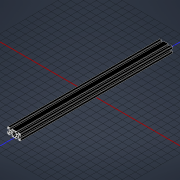
# Autodesk Inventor part: Extrusion_20x40x470
Saved by Autodesk Inventor 2022 (Build 260153000, 153)
## iProperties
Created: 2022-03-06
Part Number: Extrusion_20x40x470
Material: Aluminium 6061
Document SubType Name: Modeling
Designer: sleib
Density: 2.7 g/cm^3
Appearance: Eloxiert - Schwarz
Author: sleib
Autodesk Inventor part; units mm, degrees
ref_plane "YZ Plane" through (0, 0, 0) normal (1, 0, 0) x (0, 1, 0)
ref_plane "XZ Plane" through (0, 0, 0) normal (0, 1, 0) x (-1, 0, 0)
ref_plane "XY Plane" through (0, 0, 0) normal (0, 0, 1) x (1, 0, 0)
sketch "Skizze1" plane through (0, 0, 0) normal (0, 0, 1) x (1, 0, 0)
  circle A0 centre (10, 0) radius 2.56
  line L0 (10.5196, 4) -> (10, 3.7)
  line L1 (14, 0.5196) -> (14, 2.9393)
  line L2 (12.9393, 4) -> (10.5196, 4)
  line L3 (13.7, 0) -> (14, 0.5196)
  line L4 (14, 2.9393) -> (17.0607, 6)
  line L5 (17.0607, 6) -> (18, 6)
  line L6 (18, 6) -> (18, 3)
  line L7 (18, 3) -> (20, 3)
  line L8 (16, 7.0607) -> (12.9393, 4)
  line L9 (13, 8) -> (16, 8)
  line L10 (16, 8) -> (16, 7.0607)
  line L11 (20, 3) -> (20, 9)
  line L12 (19, 10) -> (13, 10)
  arc A1 (20, 9) -> (19, 10) centre (19, 9) ccw
  line L13 (13, 10) -> (13, 8)
  line L14 (10, 0) -> (19.7071, 9.7071) construction
  line L15 (-14.2899, 0) -> (14.2899, 0) construction
  line L16 (10, -14.2899) -> (10, 14.2899) construction
  line L17 (-28.2899, 0) -> (28.2899, 0) construction
  line L18 (0, -20.0059) -> (0, 20.0059) construction
  line L19 (14, -0.5196) -> (14, -2.9393)
  line L20 (13.7, 0) -> (14, -0.5196)
  circle A2 centre (10, 0) radius 2.56
  line L21 (10.5196, -4) -> (10, -3.7)
  line L22 (12.9393, -4) -> (10.5196, -4)
  line L23 (17.0607, -6) -> (18, -6)
  line L24 (14, -2.9393) -> (17.0607, -6)
  line L25 (16, -8) -> (16, -7.0607)
  line L26 (13, -8) -> (16, -8)
  line L27 (10, 0) -> (19.7071, -9.7071) construction
  line L28 (20, -3) -> (20, -9)
  line L29 (19, -10) -> (13, -10)
  arc A3 (19, -10) -> (20, -9) centre (19, -9) ccw
  line L30 (13, -10) -> (13, -8)
  line L31 (16, -7.0607) -> (12.9393, -4)
  line L32 (18, -3) -> (20, -3)
  line L33 (18, -6) -> (18, -3)
  line L34 (-14, 0.5196) -> (-14, 2.9393)
  line L35 (-13.7, 0) -> (-14, 0.5196)
  circle A4 centre (-10, 0) radius 2.56
  line L36 (-10.5196, 4) -> (-10, 3.7)
  line L37 (-12.9393, 4) -> (-10.5196, 4)
  line L38 (-17.0607, 6) -> (-18, 6)
  line L39 (-14, 2.9393) -> (-17.0607, 6)
  line L40 (-16, 8) -> (-16, 7.0607)
  line L41 (-13, 8) -> (-16, 8)
  line L42 (-10, 0) -> (-19.7071, 9.7071) construction
  line L43 (-10, -14.2899) -> (-10, 14.2899) construction
  line L44 (-20, 3) -> (-20, 9)
  line L45 (-19, 10) -> (-13, 10)
  arc A5 (-19, 10) -> (-20, 9) centre (-19, 9) ccw
  line L46 (-13, 10) -> (-13, 8)
  line L47 (-16, 7.0607) -> (-12.9393, 4)
  line L48 (-18, 3) -> (-20, 3)
  line L49 (-18, 6) -> (-18, 3)
  line L50 (-13.7, 0) -> (-14, -0.5196)
  line L51 (-14, -0.5196) -> (-14, -2.9393)
  line L52 (-10.5196, -4) -> (-10, -3.7)
  circle A6 centre (-10, 0) radius 2.56
  line L53 (-12.9393, -4) -> (-10.5196, -4)
  line L54 (-13, -10) -> (-13, -8)
  line L55 (-16, -7.0607) -> (-12.9393, -4)
  line L56 (-16, -8) -> (-16, -7.0607)
  line L57 (-13, -8) -> (-16, -8)
  line L58 (-14, -2.9393) -> (-17.0607, -6)
  line L59 (-10, 0) -> (-19.7071, -9.7071) construction
  line L60 (-19, -10) -> (-13, -10)
  line L61 (-17.0607, -6) -> (-18, -6)
  arc A7 (-20, -9) -> (-19, -10) centre (-19, -9) ccw
  line L62 (-20, -3) -> (-20, -9)
  line L63 (-18, -3) -> (-20, -3)
  line L64 (-18, -6) -> (-18, -3)
  line L65 (-9.4804, 4) -> (-10, 3.7)
  line L66 (-7.0607, -4) -> (-9.4804, -4)
  line L67 (-9.4804, -4) -> (-10, -3.7)
  line L68 (-7.0607, 4) -> (-9.4804, 4)
  line L69 (-4, 8) -> (-4, 7.0607)
  line L70 (-7, 8) -> (-4, 8)
  line L71 (-1, 10) -> (-7, 10)
  line L72 (-7, 10) -> (-7, 8)
  line L73 (-4, -7.0607) -> (-7.0607, -4)
  line L74 (-4, -8) -> (-4, -7.0607)
  line L75 (-1, -10) -> (-7, -10)
  line L76 (-7, -8) -> (-4, -8)
  line L77 (-7, -10) -> (-7, -8)
  line L78 (-4, 7.0607) -> (-7.0607, 4)
  line L79 (9.4804, 4) -> (10, 3.7)
  line L80 (7.0607, 4) -> (9.4804, 4)
  line L81 (4, 8) -> (4, 7.0607)
  line L82 (7, 8) -> (4, 8)
  line L83 (1, 10) -> (7, 10)
  line L84 (7, 10) -> (7, 8)
  line L85 (4, 7.0607) -> (7.0607, 4)
  line L86 (9.4804, -4) -> (10, -3.7)
  line L87 (7.0607, -4) -> (9.4804, -4)
  line L88 (7, -10) -> (7, -8)
  line L89 (4, -7.0607) -> (7.0607, -4)
  line L90 (4, -8) -> (4, -7.0607)
  line L91 (7, -8) -> (4, -8)
  line L92 (1, -10) -> (7, -10)
  line L93 (-1, 10) -> (1, 10)
  line L94 (-1, -10) -> (1, -10)
  line L95 (2.9393, 8) -> (-2.9393, 8)
  line L96 (2.9393, 8) -> (2.9393, 6)
  line L97 (6, 0.5196) -> (6, 2.9393)
  line L98 (6.3, 0) -> (6, 0.5196)
  line L99 (6, 2.9393) -> (2.9393, 6)
  line L100 (6.3, 0) -> (6, -0.5196)
  line L101 (6, -0.5196) -> (6, -2.9393)
  line L102 (6, -2.9393) -> (2.9393, -6)
  line L103 (-6.3, 0) -> (-6, -0.5196)
  line L104 (-6, 2.9393) -> (-2.9393, 6)
  line L105 (-6, 0.5196) -> (-6, 2.9393)
  line L106 (-6.3, 0) -> (-6, 0.5196)
  line L107 (-6, -0.5196) -> (-6, -2.9393)
  line L108 (-6, -2.9393) -> (-2.9393, -6)
  line L109 (-2.9393, 8) -> (-2.9393, 6)
  line L110 (2.9393, -6) -> (2.9393, -8)
  line L111 (2.9393, -8) -> (-2.9393, -8)
  line L112 (-2.9393, -8) -> (-2.9393, -6)
  point P0 (0, 0)
  point P1 (0, 8)
  dimension "d2" = 1.5
  dimension "d3" = 3
  dimension "d4" = 4
  dimension "d5" = 0.3
  dimension "d6" = 2
  dimension "d7" = 6
  dimension "d8" = 10
  dimension "d9" = 10
  dimension "d10" = 2
  dimension "d11" = 3
  dimension "d12" = 6
  dimension "d13" = 1
  dimension "d14" = 4
  dimension "d15" = 0.3
  dimension "d16" = 0.5196
  dimension "d17" = 0.5196
  dimension "d18" = 5.12
  dimension "d20" = 20
  constraints: 222 end point, 98 symmetric about line, 10 point on line, 9 point on circle, 8 centre point, 8 perpendicular, 4 coincident, 3 collinear, 3 vertical, 2 horizontal, 2 tangent, 1 midpoint, 7 other
  measures "d2" distance between parallel lines of L4 L8
  measures "d3" distance between parallel lines of L7 L15
  measures "d4" distance between parallel lines of L6 L1
  measures "d5" distance from line of L3.start L1
  measures "d6" distance between parallel lines of L11 L6
  measures "d7" distance between parallel lines of L15 L5
  measures "d8" distance between parallel lines of L11 L16
  measures "d9" distance between parallel lines of L15 L12
  measures "d10" distance between parallel lines of L9 L12
  measures "d11" distance between parallel lines of L13 L16
  measures "d12" distance between parallel lines of L10 L16
  measures "d13" radius of A1
  measures "d14" distance between parallel lines of L2 L9
  measures "d15" distance from line of L2 L0.end
  measures "d16" horizontal distance of L0.start L0.end
  measures "d17" vertical distance of L3.start L1.start
  measures "d18" diameter of A0
  measures "d20" distance between parallel lines of L11 L18
extrude "Extrusion1" add sketch "Skizze1" along normal mid plane 470
